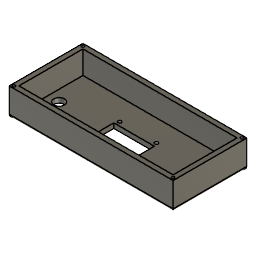
case (Autodesk Fusion 360 design; units mm, degrees)
part number: 2026-06-01-17-49-24-665
Autodesk Fusion 360 part; units mm, degrees
sketch "Sketch1" plane through (0, 0, 0) normal (0, 0, 1) x (1, 0, 0)
  line L0 (-12.5281, 6.3856) -> (12.1719, 6.3856)
  line L1 (12.1719, 6.3856) -> (12.1719, -4.8144)
  line L2 (12.1719, -4.8144) -> (-12.5281, -4.8144)
  line L3 (-12.5281, -4.8144) -> (-12.5281, 6.3856)
  circle A0 centre (40.3, 0.7856) radius 3.25
  circle A1 centre (-40.3, 0.7856) radius 3.25
  line L4 (-50, 25) -> (50, 25)
  line L5 (50, 25) -> (50, -20)
  line L6 (50, -20) -> (-50, -20)
  line L7 (-50, -20) -> (-50, 25)
  dimension "d1" = 11.2
  dimension "d2" = 24.7
  dimension "d3" = 6.5
  dimension "d4" = 40.3
  dimension "d5" = 6.5
  dimension "d6" = 40.3
  constraint horizontal L0
  constraint vertical L1
  constraint horizontal L2
  constraint vertical L3
  constraint horizontal L4
  constraint vertical L5
  constraint horizontal L6
  constraint vertical L7
  measures "d1" distance of L0.start L2.end
  measures "d2" distance of L0.start L0.end
  measures "d3" diameter of A0
  measures "d4" horizontal distance of origin A0.centre
  measures "d5" diameter of A1
  measures "d6" horizontal distance of origin A1.centre
extrude "Extrude1" add sketch "Sketch1" along normal blind 5
extrude "Extrude2" add sketch "Sketch1" along normal blind 10 thin wall 3 on the right open curves L6 L7 L4 L5
fillet "Fillet1" radius 2 4 edges at (-50, 2.5, 0) (0, -20, 0) (0, 25, 0) (50, 2.5, 0)
extrude "Extrude3" cut 1 faces at (-4.176, 16.7952, 5) along direction (0, 0, -1) blind 3
extrude "Extrude4" add 1 faces at (-15.6667, 24, 10) along direction (0, 0, 1) blind 7
sketch "Sketch2" plane through (0, 0, 2) normal (0, 0, 1) x (-1, 0, 0)
  line L0 (47, -22) -> (47, 17)
  line L1 (47, 17) -> (-47, 17)
  line L2 (-47, 17) -> (-47, -22)
  line L3 (-47, -22) -> (47, -22)
  circle A0 centre (40.3, -0.7856) radius 3.25
  line L4 (-12.1719, 4.8144) -> (12.5281, 4.8144)
  line L5 (12.5281, 4.8144) -> (12.5281, -6.3856)
  line L6 (12.5281, -6.3856) -> (-12.1719, -6.3856)
  line L7 (-12.1719, -6.3856) -> (-12.1719, 4.8144)
  circle A1 centre (-40.3, -0.7856) radius 3.25
  line L8 (13.1345, -10.9356) -> (-12.8655, -10.9356)
  line L9 (-12.8655, -10.9356) -> (-12.8655, 15.0644)
  line L10 (-12.8655, 15.0644) -> (13.1345, 15.0644)
  line L11 (13.1345, 15.0644) -> (13.1345, -10.9356)
  circle A2 centre (11.3345, -8.7356) radius 1.25
  circle A3 centre (-11.0655, -8.7356) radius 1.25
  circle A4 centre (11.3345, 13.1644) radius 1.25
  circle A5 centre (-11.0655, 13.1644) radius 1.25
  line L12 (12.5281, -6.3856) -> (-12.1719, -6.3856)
  dimension "d18" = 26
  dimension "d19" = 26
  dimension "d20" = 2.5
  dimension "d21" = 2.2
  dimension "d22" = 1.8
  dimension "d23" = 2.5
  dimension "d24" = 1.8
  dimension "d25" = 2.2
  dimension "d26" = 2.5
  dimension "d27" = 1.8
  dimension "d28" = 1.9
  dimension "d29" = 2.5
  dimension "d30" = 1.9
  dimension "d31" = 1.8
  dimension "d33" = 4.55
  constraint horizontal L8
  constraint vertical L9
  constraint horizontal L10
  constraint vertical L11
  measures "d18" distance of L8.start L10.end
  measures "d19" distance of L8.start L8.end
  measures "d20" diameter of A2
  measures "d21" distance of L8 A2.centre
  measures "d22" distance of L11 A2.centre
  measures "d23" diameter of A3
  measures "d24" distance of L9 A3.centre
  measures "d25" distance of L8 A3.centre
  measures "d26" diameter of A4
  measures "d27" distance of L11 A4.centre
  measures "d28" distance of L10 A4.centre
  measures "d29" diameter of A5
  measures "d30" distance of L10 A5.centre
  measures "d31" distance of L9 A5.centre
  measures "d33" distance of L8 L12
extrude "Extrude5" cut sketch "Sketch2" against normal blind 1 contours A2 | A3 | A4 | A5
extrude "Extrude6" add sketch "Sketch2" along normal blind 1 contours L0 L1 L2 L3
extrude "Extrude7" add 1 faces at (-3.5526, -7.3631, 2) along direction (0, 0, 1) blind 1
thread "Thread1" "ISO Metric profile 2.5 M2.5x0.45 M2.5x0.45 6H" major diameter 2.58 minor diameter 2.0755 pitch 0.45 angle 60 resizes the face on face at (-12.5829, 8.7979, 2.3333)
thread "Thread2" "ISO Metric profile 2.5 M2.5x0.45 M2.5x0.45 6H" major diameter 2.58 minor diameter 2.0755 pitch 0.45 angle 60 resizes the face on face at (9.8171, 8.7979, 2.3333)
thread "Thread3" "ISO Metric profile 2.5 M2.5x0.45 M2.5x0.45 6H" major diameter 2.58 minor diameter 2.0755 pitch 0.45 angle 60 resizes the face on face at (9.8171, -13.1021, 2.3333)
thread "Thread4" "ISO Metric profile 2.5 M2.5x0.45 M2.5x0.45 6H" major diameter 2.58 minor diameter 2.0755 pitch 0.45 angle 60 resizes the face on face at (-12.5829, -13.1021, 2.3333)
sketch "Sketch3" plane through (0, 0, 3) normal (0, 0, 1) x (-1, 0, 0)
  line L0 (-12.1719, 4.8144) -> (12.5281, 4.8144)
  line L1 (12.5281, 4.8144) -> (12.5281, -6.3856)
  line L2 (12.5281, -6.3856) -> (-12.1719, -6.3856)
  line L3 (-12.1719, -6.3856) -> (-12.1719, 4.8144)
  circle A0 centre (11.3345, -8.7356) radius 1.0377
  circle A1 centre (11.3345, 13.1644) radius 1.0377
  circle A2 centre (-11.0655, -8.7356) radius 1.0377
  circle A3 centre (-11.0655, 13.1644) radius 1.0377
  circle A4 centre (40.3, -0.7856) radius 3.25
  circle A5 centre (-40.3, -0.7856) radius 3.25
  line L4 (-47, -22) -> (47, -22)
  line L5 (47, -22) -> (47, 17)
  line L6 (47, 17) -> (-47, 17)
  line L7 (-47, 17) -> (-47, -22)
sketch "Sketch4" plane through (0, 0, 3) normal (0, 0, 1) x (-1, 0, 0)
  line L0 (32.5206, -8.7687) -> (14.5206, -8.7687)
  line L1 (14.5206, -8.7687) -> (14.5206, 13.7313)
  line L2 (14.5206, 13.7313) -> (32.5206, 13.7313)
  line L3 (32.5206, 13.7313) -> (32.5206, -8.7687)
  dimension "d50" = 22.5
  dimension "d51" = 18
  constraint horizontal L0
  constraint vertical L1
  constraint horizontal L2
  constraint vertical L3
  measures "d50" distance of L0.start L2.end
  measures "d51" distance of L0.start L0.end
sketch "Sketch5" plane through (0, 0, 0) normal (0, 0, -1) x (1, 0, 0)
  circle A0 centre (40.3, -0.7856) radius 3.25
  line L0 (-12.5281, 4.8144) -> (12.1719, 4.8144)
  line L1 (12.1719, 4.8144) -> (12.1719, -6.3856)
  line L2 (12.1719, -6.3856) -> (-12.5281, -6.3856)
  line L3 (-12.5281, -6.3856) -> (-12.5281, 4.8144)
  circle A1 centre (-40.3, -0.7856) radius 3.25
  line L4 (48, -23) -> (48, 18)
  line L5 (48, 18) -> (-48, 18)
  line L6 (-48, 18) -> (-48, -23)
  line L7 (-48, -23) -> (48, -23)
  line L8 (29.0858, 10) -> (28, 10)
  line L9 (28, 10) -> (28, 8.0434)
  line L10 (27, 10) -> (26.9716, 8.0517)
  line L11 (27.8165, 6.627) -> (27.5996, 6.6322)
  line L12 (28.0873, 6.1203) -> (28.0366, 4.0258)
  line L13 (28.0366, 4.0258) -> (29.1035, 4)
  line L14 (27, 10) -> (25.8642, 10)
  arc A2 (25.8649, 8.6254) -> (27.8165, 6.627) centre (27.8649, 8.6264) ccw
  arc A3 (26.9716, 8.0517) -> (27.4675, 7.5444) centre (27.4715, 8.0444) ccw
  arc A4 (27.4675, 7.5444) -> (28, 8.0434) centre (27.5, 8.0434) ccw
  arc A5 (28.0873, 6.1203) -> (27.5996, 6.6322) centre (27.5874, 6.1324) ccw
  line L15 (25.8649, 8.6254) -> (25.8642, 10)
  line L16 (29.1035, 4) -> (29.0858, 10)
  line L17 (24, 3) -> (31, 3)
  line L18 (31, 3) -> (31, 11)
  line L19 (31, 11) -> (24, 11)
  line L20 (24, 11) -> (24, 3)
  dimension "d52" = 2
  dimension "d53" = 0.5
  constraint horizontal L8
  constraint perpendicular L8 L9
  constraint perpendicular L11 L12
  constraint perpendicular L12 L13
  constraint tangent L11 A2
  constraint tangent L10 A3
  constraint tangent L9 A4
  constraint equal A3 A4
  constraint tangent L11 A5
  constraint tangent L12 A5
  constraint equal A3 A5
  constraint tangent A2 L15
  constraint horizontal L17
  constraint vertical L18
  constraint horizontal L19
  constraint vertical L20
  measures "d52" radius of A2
  measures "d53" radius of A3
extrude "Extrude8" cut sketch "Sketch5" against normal blind 0.5 contours L17 L18 L19 L20
sketch "Sketch6" plane through (0, 0, 0) normal (0, 0, -1) x (1, 0, 0)
  line L0 (48, -23) -> (48, 18)
  line L1 (48, 18) -> (-48, 18)
  line L2 (-48, 18) -> (-48, -23)
  line L3 (-48, -23) -> (48, -23)
  circle A0 centre (-40.3, -0.7856) radius 3.25
  line L4 (-12.5281, 4.8144) -> (12.1719, 4.8144)
  line L5 (12.1719, 4.8144) -> (12.1719, -6.3856)
  line L6 (12.1719, -6.3856) -> (-12.5281, -6.3856)
  line L7 (-12.5281, -6.3856) -> (-12.5281, 4.8144)
  circle A1 centre (40.3, -0.7856) radius 3.25
  line L8 (31, 3) -> (24, 3)
  line L9 (24, 3) -> (24, 11)
  line L10 (24, 11) -> (31, 11)
  line L11 (31, 11) -> (31, 3)
  line L12 (12.8516, -11.4737) -> (-16.6364, -11.4737) construction
  line L13 (-16.6364, -11.4737) -> (-16.6364, -18.5155) construction
  line L14 (-16.6364, -18.5155) -> (12.8516, -18.5155) construction
  line L15 (12.8516, -18.5155) -> (12.8516, -11.4737) construction
  dimension "d56" = 3
sketch "Sketch7" plane through (0, 0, 17) normal (0, 0, 1) x (-1, 0, 0)
  line L0 (47, 17) -> (47, -22)
  line L1 (47, -22) -> (-47, -22)
  line L2 (-47, -22) -> (-47, 17)
  line L3 (-47, 17) -> (47, 17)
  line L4 (50, 20) -> (-50, 20)
  line L5 (-50, 20) -> (-50, -25)
  line L6 (-50, -25) -> (50, -25)
  line L7 (50, -25) -> (50, 20)
  circle A0 centre (48.5, 18.5) radius 1
  circle A1 centre (48.5, -23.5) radius 1
  circle A2 centre (-48.5, -23.5) radius 1
  circle A3 centre (-48.5, 18.5) radius 1
  dimension "d58" = 1.5
  dimension "d59" = 1.5
  dimension "d60" = 2
  dimension "d61" = 1.5
  dimension "d62" = 1.5
  dimension "d63" = 2
  dimension "d64" = 1.5
  dimension "d65" = 1.5
  dimension "d66" = 2
  dimension "d67" = 1.5
  dimension "d68" = 1.5
  measures "d58" distance of L7 A0.centre
  measures "d59" distance of L4 A0.centre
  measures "d60" diameter of A1
  measures "d61" distance of L7 A1.centre
  measures "d62" distance of L6 A1.centre
  measures "d63" diameter of A2
  measures "d64" distance of L6 A2.centre
  measures "d65" distance of L5 A2.centre
  measures "d66" diameter of A3
  measures "d67" distance of L4 A3.centre
  measures "d68" distance of L5 A3.centre
extrude "Extrude9" cut sketch "Sketch7" against normal blind 2 contours A0 | A1 | A2 | A3
thread "Thread5" "ISO Metric profile 2.0 M2x0.4 M2x0.4 6H" major diameter 2.074 minor diameter 1.623 pitch 0.4 angle 60 resizes the face on face at (47.5785, -18.8884, 15.6667)
thread "Thread6" "ISO Metric profile 2.0 M2x0.4 M2x0.4 6H" major diameter 2.074 minor diameter 1.623 pitch 0.4 angle 60 resizes the face on face at (47.5785, 23.1116, 15.6667)
thread "Thread7" "ISO Metric profile 2.0 M2x0.4 M2x0.4 6H" major diameter 2.074 minor diameter 1.623 pitch 0.4 angle 60 resizes the face on face at (-49.1617, 22.7502, 15.6667)
thread "Thread8" "ISO Metric profile 2.0 M2x0.4 M2x0.4 6H" major diameter 2.074 minor diameter 1.623 pitch 0.4 angle 60 resizes the face on face at (-48.6243, -19.4922, 15.6667)
equation "d57 = 'etch a sketch'"
